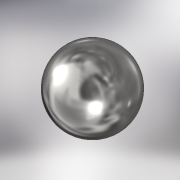
# Autodesk Inventor part: CouplerBall
Saved by Autodesk Inventor 2022.1 (Build 261234020, 234B)
## iProperties
Created: 2022-04-18
Part Number: CouplerBall
Material: Stainless Steel
Document SubType Name: Modeling
Designer: Remo
Density: 8 g/cm^3
Appearance: Semi-Polished
Author: Remo
Autodesk Inventor part; units mm, degrees
ref_plane "YZ Plane" through (0, 0, 0) normal (1, 0, 0) x (0, 1, 0)
ref_plane "XZ Plane" through (0, 0, 0) normal (0, 1, 0) x (-1, 0, 0)
ref_plane "XY Plane" through (0, 0, 0) normal (0, 0, 1) x (1, 0, 0)
sketch "Sketch1" plane through (0, 0, 0) normal (1, 0, 0) x (0, 1, 0)
  circle A0 centre (0, 0) radius 5
  line L0 (2.5, -4.3301) -> (-2.5, -4.3301)
  line L1 (0, 5) -> (0, -4.3301)
  dimension "d0" = 10
  dimension "d1" = 5
  constraints: 4 end point, 3 point on circle, 1 centre point, 1 coincident, 1 horizontal, 1 midpoint
  measures "d0" diameter of A0
  measures "d1" distance of L0.start L0.end
revolve "Revolution1" add sketch "Sketch1" angle 360 about axis through (0, 0, 5) along (0, 0, -1) picked at (0.3709, 1.8482) contours A0 L0 L1
body "Solid1"
